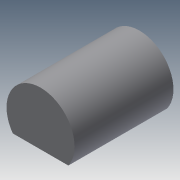
# Autodesk Inventor part: speaker_body
Saved by Autodesk Inventor 2015 (Build 190159000, 159)
## iProperties
Created: 2018-01-22
Part Number: speaker_body
Material: Generic
Document SubType Name: Modeling
Designer: rissa
Density: 1 g/cm^3
Appearance: Default
Author: rissa
Autodesk Inventor part; units mm, degrees
ref_plane "YZ Plane" through (0, 0, 0) normal (1, 0, 0) x (0, 1, 0)
ref_plane "XZ Plane" through (0, 0, 0) normal (0, 1, 0) x (-1, 0, 0)
ref_plane "XY Plane" through (0, 0, 0) normal (0, 0, 1) x (1, 0, 0)
sketch "Sketch1" plane through (0, 0, 0) normal (0, 0, 1) x (1, 0, 0)
  circle A0 centre (0, 0) radius 27.5
  dimension "d0" = 55
  constraints: 1 centre point, 1 coincident
  measures "d0" diameter of A0
extrude "Extrusion1" add sketch "Sketch1" along normal blind 80
sketch "Sketch2" plane through (0, 0, 80) normal (0, 0, 1) x (1, 0, 0)
  circle A0 centre (0, 0) radius 27.5 projected
  line L0 (-22.5, -15.8114) -> (22.5, -15.8114)
  dimension "d5" = 45
  constraints: 2 end point, 2 point on circle, 1 horizontal
  measures "d5" distance of L0.start L0.end
extrude "Extrusion2" cut sketch "Sketch2" against normal blind 80 contours L0 A0 picked at (-6.0353, -17.4405)
sketch "Sketch3" plane through (-22.5, -15.8114, 80) normal (0, -1, 0) x (1, 0, 0)
  circle A0 centre (22.5, -50) radius 20
  point P0 (22.5, -80)
  dimension "d8" = 40
  dimension "d9" = 30
  constraints: 1 centre point
  measures "d8" diameter of A0
  measures "d9" distance of point (22.5, -80) A0.centre
extrude "Extrusion3" cut sketch "Sketch3" against normal blind 30
sketch "Sketch4" plane through (0, 0, 0) normal (0, 0, -1) x (-1, 0, 0)
  arc A0 (22.5, -15.8114) -> (-22.5, -15.8114) centre (0, 0) ccw projected
  circle A1 centre (0, 0) radius 25
  line L0 (21.4678, -12.8114) -> (-21.4678, -12.8114)
  line L1 (-22.5, -15.8114) -> (22.5, -15.8114) projected
  dimension "d12" = 50
  dimension "d13" = 3
  constraints: 2 end point, 2 point on circle, 1 centre point, 1 coincident, 1 horizontal
  measures "d12" diameter of A1
  measures "d13" distance between parallel lines of L0 L1
extrude "Extrusion4" cut sketch "Sketch4" against normal blind 77 contours L0 A1
body "Solid1"
